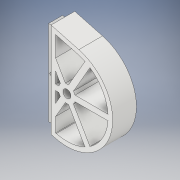
# Autodesk Inventor part: Riser Base
Saved by Autodesk Inventor 2017 SP1 (Build 210196100, 196)
## iProperties
Created: 2017-07-19
Part Number: Riser Base
Material: ABS Plastic
Document SubType Name: Modeling
Designer: zallen
Density: 1.06 g/cm^3
Appearance: CR White
Author: zallen
Autodesk Inventor part; units mm, degrees
ref_plane "YZ Plane" through (0, 0, 0) normal (1, 0, 0) x (0, 1, 0)
ref_plane "XZ Plane" through (0, 0, 0) normal (0, 1, 0) x (-1, 0, 0)
ref_plane "XY Plane" through (0, 0, 0) normal (0, 0, 1) x (1, 0, 0)
sketch "Sketch1" plane through (0, 0, 0) normal (0, 0, 1) x (1, 0, 0)
  line L0 (0, 0) -> (160, 0)
  line L1 (160, 0) -> (118.589, -154.5481) construction
  line L2 (0, 0) -> (41.411, -154.5481) construction
  line L3 (41.411, -154.5481) -> (118.589, -154.5481)
  circle A0 centre (235.8871, -103.156) radius 80 construction
  line L4 (160, 0) -> (256.5926, -25.8819)
  line L5 (118.589, -154.5481) -> (215.1815, -180.43)
  arc A1 (215.1815, -180.43) -> (256.5926, -25.8819) centre (235.8871, -103.156) ccw
  circle A2 centre (-75.8871, -103.156) radius 80 construction
  line L6 (0, 0) -> (-96.5926, -25.8819)
  line L7 (41.411, -154.5481) -> (-55.1815, -180.43)
  arc A3 (-96.5926, -25.8819) -> (-55.1815, -180.43) centre (-75.8871, -103.156) ccw
  dimension "d0" = 160
  dimension "d1" = 160
  dimension "d2" = 160
  dimension "d3" = 75
  dimension "d4" = 75
  dimension "d5" = 160
  dimension "d6" = 100
  dimension "d7" = 160
  dimension "d9" = 100
  constraints: 16 end point, 8 point on circle, 8 tangent, 4 centre point, 2 concentric, 2 parallel, 1 horizontal
  measures "d0" distance of L0.start L0.end
  measures "d1" distance of L0.end L1.end
  measures "d2" distance of L0.start L2.end
  measures "d3" angle of L0 L2
  measures "d4" angle of L0 L1
  measures "d5" diameter of A0
  measures "d6" distance of L0.end L4.end
  measures "d7" diameter of A2
  measures "d9" distance of L0.start L6.end
extrude "Extrusion1" add sketch "Sketch1" along normal blind 41.5
sketch "Sketch2" plane through (0, 0, 41.5) normal (0, 0, 1) x (1, 0, 0)
  line L0 (-26.5, -133) -> (186.5, -133)
  line L1 (186.5, -133) -> (186.5, -20)
  line L2 (186.5, -20) -> (-26.5, -20)
  line L3 (-26.5, -20) -> (-26.5, -133)
  line L4 (160, 0) -> (0, 0) projected
  point P0 (80, -20)
  point P1 (80, 0)
  dimension "d12" = 213
  dimension "d13" = 113
  dimension "d14" = 20
  constraints: 8 end point, 2 midpoint, 2 parallel, 1 horizontal, 1 perpendicular, 1 vertical alignment
  measures "d12" distance of L2.end L1.end
  measures "d13" distance of L1.end L0.end
  measures "d14" distance between parallel lines of L4 L2
extrude "Extrusion2" cut sketch "Sketch2" against normal through all
sketch "Sketch3" plane through (0, 0, 41.5) normal (0, 0, 1) x (1, 0, 0)
  line L0 (-26.5, -133) -> (-26.5, -20) construction
  line L1 (-26.5, -20) -> (186.5, -20) construction
  line L2 (186.5, -20) -> (186.5, -133) construction
  line L3 (186.5, -133) -> (-26.5, -133) construction
  line L4 (-48.0481, 1.5481) -> (-48.0481, -154.5481) construction
  line L5 (-48.0481, -154.5481) -> (208.0481, -154.5481) construction
  line L6 (208.0481, -154.5481) -> (208.0481, 1.5481) construction
  line L7 (208.0481, 1.5481) -> (-48.0481, 1.5481) construction
  line L8 (41.411, -154.5481) -> (118.589, -154.5481) construction
  line L9 (-48.0481, 1.5481) -> (-48.0481, -178.5186) construction
  line L10 (-55.1815, -180.43) -> (41.411, -154.5481) construction
  line L11 (208.0481, 1.5481) -> (208.0481, -178.5186) construction
  line L12 (118.589, -154.5481) -> (215.1815, -180.43) construction
  line L13 (-48.0481, -178.5186) -> (208.0481, -178.5186) construction
  line L14 (-48.0481, 1.5481) -> (208.0481, 1.5481) construction
  line L15 (160, 0) -> (256.5926, -25.8819) construction
  line L16 (208.2963, -12.941) -> (208.0481, -178.5186)
  line L17 (208.2963, -12.941) -> (256.5926, -25.8819)
  line L18 (208.0481, -178.5186) -> (215.1815, -180.43)
  arc A0 (215.1815, -180.43) -> (256.5926, -25.8819) centre (235.8871, -103.156) ccw
  line L19 (208.0481, 1.5481) -> (-166.9519, 1.5481)
  line L20 (-166.9519, 1.5481) -> (-166.9519, -188.4519)
  line L21 (-166.9519, -188.4519) -> (208.0481, -188.4519)
  line L22 (208.0481, -188.4519) -> (208.0481, 1.5481)
  point P0 (0, 0)
  point P1 (80, -154.5481)
  dimension "d17" = 190
  dimension "d18" = 375
  constraints: 30 end point, 3 midpoint, 3 parallel, 3 perpendicular, 2 point on circle, 2 point on line, 2 tangent, 2 vertical, 1 centre point, 1 collinear, 1 horizontal, 3 other
  measures "d17" distance of L19.end L20.end
  measures "d18" distance of L20.end L21.end
extrude "Extrusion3" cut sketch "Sketch3" against normal through all contours L22 L21 L20 L19
sketch "Sketch4" plane through (0, 0, 41.5) normal (0, 0, 1) x (1, 0, 0)
  arc A0 (215.1815, -180.43) -> (256.5926, -25.8819) centre (235.8871, -103.156) ccw projected
  circle A1 centre (235.8871, -103.156) radius 7
  point P0 (0, 0)
  dimension "d21" = 14
  constraints: 1 centre point, 1 coincident
  measures "d21" diameter of A1
extrude "Extrusion4" cut sketch "Sketch4" against normal through all
sketch "Sketch5" plane through (208.0481, -178.5186, 41.5) normal (-1, 0, 0) x (0, 0, 1)
  line L0 (-41.5, 165.6442) -> (0, 165.6442) projected
  line L1 (-41.5, 0) -> (-41.5, 165.6442) projected
  line L2 (0, 0) -> (-41.5, 0) projected
  line L3 (0, 165.6442) -> (0, 0) projected
  line L4 (-33, 157.1442) -> (-8.5, 157.1442)
  line L5 (-8.5, 157.1442) -> (-8.5, 8.5)
  line L6 (-8.5, 8.5) -> (-33, 8.5)
  line L7 (-33, 8.5) -> (-33, 157.1442)
  point P0 (-41.5, 178.5186)
  dimension "d24" = 8.5
  constraints: 8 end point, 3 other
  measures "d24" distance between parallel lines of L1 L7
extrude "Extrusion5" add sketch "Sketch5" along normal blind 13 contours L4 L5 L6 L7
sketch "Sketch6" plane through (208.0481, -170.0186, 8.5) normal (0, 0, -1) x (-1, 0, 0)
  circle A0 centre (8, 74.3221) radius 2.5
  line L0 (0, -8.5) -> (0, 157.1442) projected
  point P0 (208.0481, 170.0186)
  point P1 (0, 74.3221)
  dimension "d27" = 5
  dimension "d28" = 8
  constraints: 1 centre point, 1 horizontal alignment, 1 midpoint
  measures "d27" diameter of A0
  measures "d28" distance from line of L0 A0.centre
extrude "Extrusion6" cut sketch "Sketch6" against normal through all
sketch "Sketch7" plane through (0, 0, 0) normal (0, 0, -1) x (-1, 0, 0)
  circle A0 centre (-235.8871, -103.156) radius 7 projected
  line L0 (-208.0481, -178.5186) -> (-208.0481, -12.8745) projected
  line L1 (-208.0481, -12.8745) -> (-256.5926, -25.8819) projected
  arc A1 (-256.5926, -25.8819) -> (-215.1815, -180.43) centre (-235.8871, -103.156) ccw projected
  line L2 (-215.1815, -180.43) -> (-208.0481, -178.5186) projected
  line L3 (-254.522, -33.6093) -> (-216.0481, -23.3003)
  line L4 (-216.0481, -23.3003) -> (-216.0481, -172.38)
  line L5 (-216.0481, -172.38) -> (-217.2521, -172.7026)
  arc A2 (-254.522, -33.6093) -> (-217.2521, -172.7026) centre (-235.8871, -103.156) ccw
  circle A3 centre (-235.8871, -103.156) radius 15
  point P0 (0, 0)
  dimension "d31" = 8
  dimension "d32" = 8
  constraints: 6 end point, 2 centre point, 2 point on circle, 3 other
  measures "d31" distance between parallel lines of L1 L3
  measures "d32" radial gap between concentric circles of A0 A3
extrude "Extrusion7" cut sketch "Sketch7" against normal through all contours L3 L4 L5 A2
sketch "Sketch8" plane through (0, 0, 0) normal (0, 0, -1) x (-1, 0, 0)
  circle A0 centre (-235.8871, -103.156) radius 7 construction
  circle A1 centre (-235.8871, -103.156) radius 15 construction
  line L0 (-235.8871, -103.156) -> (-159.7277, -103.156) construction
  line L1 (-221.7449, -98.156) -> (-123.6167, -98.156) construction
  line L2 (-221.7449, -108.156) -> (-123.6167, -108.156) construction
  line L3 (-233.1461, -88.4085) -> (-184.082, -3.427) construction
  line L4 (-224.4859, -93.4085) -> (-175.4217, -8.427) construction
  line L5 (-247.2883, -93.4085) -> (-296.3524, -8.427) construction
  line L6 (-238.628, -88.4085) -> (-287.6921, -3.427) construction
  line L7 (-250.0292, -108.156) -> (-348.1575, -108.156) construction
  line L8 (-250.0292, -98.156) -> (-348.1575, -98.156) construction
  line L9 (-238.628, -117.9034) -> (-287.6921, -202.885) construction
  line L10 (-247.2883, -112.9034) -> (-296.3524, -197.885) construction
  line L11 (-224.4859, -112.9034) -> (-175.4217, -197.885) construction
  line L12 (-233.1461, -117.9034) -> (-184.082, -202.885) construction
  line L13 (-216.0481, -23.3003) -> (-216.0481, -172.38) construction
  arc A2 (-254.522, -33.6093) -> (-217.2521, -172.7026) centre (-235.8871, -103.156) ccw construction
  line L14 (-254.522, -33.6093) -> (-216.0481, -23.3003) construction
  line L15 (-216.0481, -172.38) -> (-217.2521, -172.7026) construction
  line L16 (-221.7449, -98.156) -> (-216.0481, -98.156)
  line L17 (-221.7449, -108.156) -> (-216.0481, -108.156)
  line L18 (-224.4859, -112.9034) -> (-216.0481, -127.518)
  line L19 (-233.1461, -117.9034) -> (-216.0481, -147.518)
  line L20 (-238.628, -117.9034) -> (-267.47, -167.8593)
  line L21 (-276.1303, -162.8593) -> (-247.2883, -112.9034)
  line L22 (-250.0292, -108.156) -> (-307.7132, -108.156)
  line L23 (-250.0292, -98.156) -> (-307.7132, -98.156)
  line L24 (-247.2883, -93.4085) -> (-276.1303, -43.4527)
  line L25 (-238.628, -88.4085) -> (-267.47, -38.4527)
  line L26 (-233.1461, -88.4085) -> (-216.0481, -58.7939)
  line L27 (-224.4859, -93.4085) -> (-216.0481, -78.7939)
  line L28 (-216.0481, -58.7939) -> (-216.0481, -78.7939)
  line L29 (-216.0481, -98.156) -> (-216.0481, -108.156)
  line L30 (-216.0481, -127.518) -> (-216.0481, -147.518)
  arc A3 (-267.47, -38.4527) -> (-276.1303, -43.4527) centre (-235.8871, -103.156) ccw
  arc A4 (-307.7132, -98.156) -> (-307.7132, -108.156) centre (-235.8871, -103.156) ccw
  arc A5 (-276.1303, -162.8593) -> (-267.47, -167.8593) centre (-235.8871, -103.156) ccw
  arc A6 (-221.7449, -108.156) -> (-221.7449, -98.156) centre (-235.8871, -103.156) ccw
  arc A7 (-233.1461, -117.9034) -> (-224.4859, -112.9034) centre (-235.8871, -103.156) ccw
  arc A8 (-247.2883, -112.9034) -> (-238.628, -117.9034) centre (-235.8871, -103.156) ccw
  arc A9 (-250.0292, -98.156) -> (-250.0292, -108.156) centre (-235.8871, -103.156) ccw
  arc A10 (-238.628, -88.4085) -> (-247.2883, -93.4085) centre (-235.8871, -103.156) ccw
  arc A11 (-224.4859, -93.4085) -> (-233.1461, -88.4085) centre (-235.8871, -103.156) ccw
  point P0 (0, 0)
  dimension "d36" = 5
  dimension "d37" = 5
  dimension "d40" = 360
  constraints: 56 end point, 26 point on circle, 20 point on line, 9 centre point, 9 concentric, 3 collinear, 3 horizontal, 37 other
  measures "d36" distance between parallel lines of L1 L0
  measures "d37" distance between parallel lines of L0 L2
extrude "Extrusion8" add sketch "Sketch8" against normal blind 41.5
body "Solid1"
